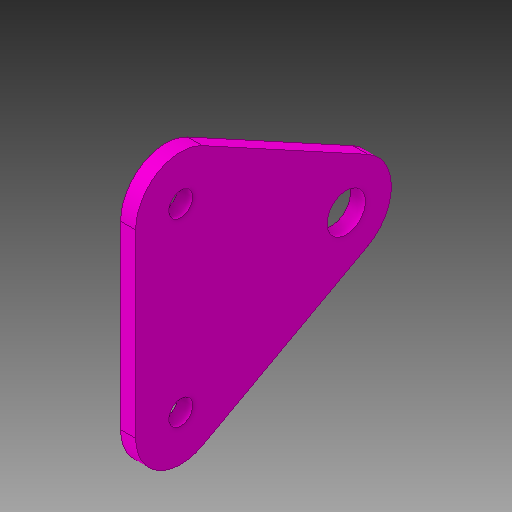
# Autodesk Inventor part: roller plate
Saved by Autodesk Inventor 2017 SP1 (Build 210196100, 196)
## iProperties
Created: 2018-01-21
Part Number: roller plate
Material: Nylon 6/6
Document SubType Name: Modeling
Designer: Ben
Density: 1.13 g/cm^3
Appearance: Magenta
Mass: 7.09902 g
Surface Area: 47.0338 cm^2
Volume: 6.28232 cm^3
Author: Ben
Autodesk Inventor part; units mm, degrees
ref_plane "YZ Plane" through (0, 0, 0) normal (1, 0, 0) x (0, 1, 0)
ref_plane "XZ Plane" through (0, 0, 0) normal (0, 1, 0) x (-1, 0, 0)
ref_plane "XY Plane" through (0, 0, 0) normal (0, 0, 1) x (1, 0, 0)
sketch "Sketch1" plane through (0, 0, 0) normal (1, 0, 0) x (0, 1, 0)
  line L0 (19.05, 0) -> (-19.05, 0) construction
  circle A0 centre (19.05, 0) radius 2.54
  circle A1 centre (-19.05, 0) radius 2.54
  circle A2 centre (0, -34.925) radius 4.064
  line L1 (0, 0) -> (0, -34.925) construction
  arc A3 (27.412, -4.5611) -> (19.05, 9.525) centre (19.05, 0) ccw
  arc A4 (-19.05, 9.525) -> (-27.412, -4.5611) centre (-19.05, 0) ccw
  arc A5 (-8.362, -39.4861) -> (8.362, -39.4861) centre (0, -34.925) ccw
  line L2 (-8.362, -39.4861) -> (-27.412, -4.5611)
  line L3 (-19.05, 9.525) -> (19.05, 9.525)
  line L4 (27.412, -4.5611) -> (8.362, -39.4861)
  dimension "d0" = 5.08
  dimension "d2" = 38.1
  dimension "d3" = 8.128
  dimension "d4" = 34.925
  dimension "d5" = 9.525
  constraints: 10 end point, 6 centre point, 6 coincident, 6 point on circle, 6 tangent, 3 equal radius, 1 horizontal, 1 midpoint, 1 vertical
  measures "d0" diameter of A0
  measures "d2" distance of L0.start L0.end
  measures "d3" diameter of A2
  measures "d4" distance from line of L0 L1.end
  measures "d5" radius of A3
extrude "Extrusion1" add sketch "Sketch1" along normal blind 3.175
body "Solid1"
